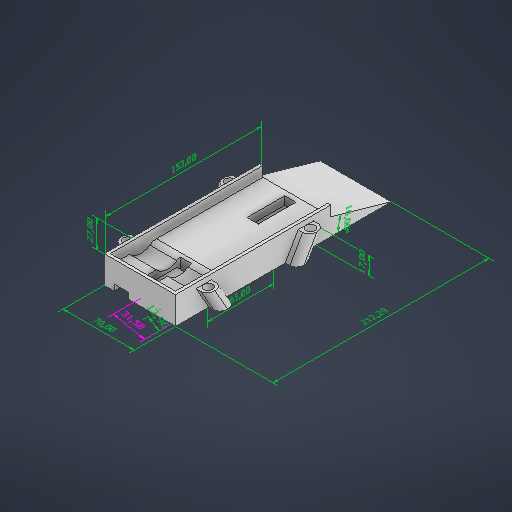
# Autodesk Inventor part: BaseCabina_v03
Saved by Autodesk Inventor 2026.1 (Build 301233020, 233B)
## iProperties
Created: 2025-10-09
Part Number: BaseCabina_v03
Material: Generic
Document SubType Name: Modeling
Designer: tito.luyo
Density: 1 g/cm^3
Appearance: Default
Author: tito.luyo
## iProperties of the stored document BaseCabina_3DPrint.ipt
Created: 2025-10-20
Part Number: BaseCabina_3DPrint
Material: Generic
Document SubType Name: Modeling
Designer: tito.luyo
Density: 1 g/cm^3
Appearance: Default
Author: tito.luyo
Autodesk Inventor part; units mm, degrees
ref_plane "YZ Plane" through (0, 0, 0) normal (1, 0, 0) x (0, 1, 0)
ref_plane "XZ Plane" through (0, 0, 0) normal (0, 1, 0) x (-1, 0, 0)
ref_plane "XY Plane" through (0, 0, 0) normal (0, 0, 1) x (1, 0, 0)
sketch "SketchBase" plane through (0, 0, 0) normal (0, 1, 0) x (-1, 0, 0)
  line L0 (0, 0) -> (70, 0)
  line L1 (70, 0) -> (70, -150)
  line L2 (70, -150) -> (0, -150)
  line L3 (0, -150) -> (0, 0)
  dimension "cabina_ancho" = 70
  dimension "cabina_largo" = 150
  constraints: 8 end point, 2 parallel, 1 horizontal, 1 perpendicular
  measures "cabina_ancho" distance of L1.end L2.end
  measures "cabina_largo" distance of L0.end L1.end
extrude "Base" add sketch "SketchBase" along normal blind 17
sketch "SketchBateria" plane through (0, 0, 0) normal (0, -1, 0) x (1, 0, 0)
  line L0 (-4, -48.5) -> (-35, -48.5)
  line L1 (-35, -48.5) -> (-35, -103.5)
  line L2 (-35, -103.5) -> (-4, -103.5)
  line L3 (-4, -103.5) -> (-4, -48.5)
  line L4 (0, 0) -> (0, -150) projected
  line L5 (-70, 0) -> (0, 0) projected
  point P0 (-19.5, -48.5)
  dimension "bateria_ancho" = 31
  dimension "bateria_largo" = 55
  dimension "bateria_sep_fondo" = 48.5
  dimension "d119" = 35
  constraints: 8 end point, 2 parallel, 1 horizontal, 1 midpoint, 1 perpendicular
  measures "bateria_ancho" distance of L2.end L1.end
  measures "bateria_largo" distance of L1.end L0.end
  measures "bateria_sep_fondo" distance from line of point (-19.5, -48.5) L5
  measures "d119" distance between parallel lines of L4 L1
extrude "Bateria" cut sketch "SketchBateria" against normal blind 7
sketch "SketchMicroControlador" plane through (0, 0, 0) normal (0, -1, 0) x (1, 0, 0)
  line L0 (-43, -5) -> (-63, -5)
  line L1 (-63, -5) -> (-63, -35)
  line L2 (-63, -35) -> (-43, -35)
  line L3 (-43, -35) -> (-43, -5)
  line L4 (-70, -150) -> (-70, 0) projected
  line L5 (-70, 0) -> (0, 0) projected
  dimension "micro_ancho" = 20
  dimension "micro_largo" = 30
  dimension "micro_sep_lateral" = 7
  dimension "micro_sep_fondo" = 5
  constraints: 8 end point, 2 parallel, 1 horizontal, 1 perpendicular
  measures "micro_ancho" distance of L2.end L1.end
  measures "micro_largo" distance of L1.end L0.end
  measures "micro_sep_lateral" distance between parallel lines of L4 L1
  measures "micro_sep_fondo" distance between parallel lines of L5 L0
extrude "MicroControlador" cut sketch "SketchMicroControlador" against normal blind 6
sketch "SketchSensorPresencia" plane through (0, 17, 0) normal (0, 1, 0) x (1, 0, 0)
  line L0 (-29.5, 108) -> (-40.5, 108)
  line L1 (-40.5, 108) -> (-40.5, 145)
  line L2 (-40.5, 145) -> (-29.5, 145)
  line L3 (-29.5, 145) -> (-29.5, 108)
  line L4 (0, 150) -> (-70, 150) projected
  line L5 (0, 0) -> (0, 150) projected
  point P0 (-35, 150)
  point P1 (-35, 145)
  dimension "presencia_ancho" = 11
  dimension "presencia_largo" = 37
  dimension "presencia_sep_fondo" = 5
  dimension "presencia_sep_lateral" = 29.5
  constraints: 8 end point, 2 midpoint, 2 parallel, 1 horizontal, 1 perpendicular
  measures "presencia_ancho" distance of L1.end L2.end
  measures "presencia_largo" distance of L0.end L1.end
  measures "presencia_sep_fondo" distance of point (-35, 150) point (-35, 145)
  measures "presencia_sep_lateral" distance between parallel lines of L5 L3
extrude "SensorPresencia" cut sketch "SketchSensorPresencia" against normal blind 8
sketch "SketchSoporte" plane through (0, 0, 0) normal (0, -1, 0) x (1, 0, 0)
  line L0 (11, -45) -> (-2, -45)
  line L1 (-2, -45) -> (-2, -30)
  line L2 (-2, -30) -> (11, -30)
  line L3 (11, -30) -> (11, -45)
  line L4 (-70, 0) -> (0, 0) projected
  line L5 (0, 0) -> (0, -150) projected
  dimension "soporte_ancho" = 13
  dimension "soporte_largo" = 15
  dimension "soporte_sep_extremo" = 30
  dimension "soporte_ins_lateral" = 11
  constraints: 8 end point, 2 parallel, 1 horizontal, 1 perpendicular
  measures "soporte_ancho" distance of L1.end L2.end
  measures "soporte_largo" distance of L0.end L1.end
  measures "soporte_sep_extremo" distance between parallel lines of L2 L4
  measures "soporte_ins_lateral" distance between parallel lines of L5 L3
sketch "SketchSoporteGuiaInclinada" plane through (0, 0, 0) normal (1, 0, 0) x (0, 0, -1)
  line L0 (150, 0) -> (0, 0) projected
  line L1 (20, 0) -> (7.2983, 22)
  dimension "soporte_guia_sep_extremo" = 20
  dimension "soporte_guia_inclinacion" = 60
  dimension "soporte_guia_altura" = 22
  constraints: 2 end point, 1 point on line
  measures "soporte_guia_sep_extremo" distance of L0.end L1.start
  measures "soporte_guia_inclinacion" angle of L0 L1
  measures "soporte_guia_altura" distance from line of L0 L1.end
sweep "Soporte" add profiles "SketchSoporte" path "SketchSoporteGuiaInclinada" path curves L1
sketch "SketchSoporteHueco" plane through (-2, 22, -17.2983) normal (0, 1, 0) x (1, 0, 0)
  circle A0 centre (6.5, 7.5) radius 4.45
  line L0 (13, 15) -> (0, 15) projected
  line L1 (0, 15) -> (0, 0) projected
  point P0 (2, -17.2983)
  dimension "soporte_hueco_diametro" = 8.9
  dimension "soporte_hueco_sep_largo" = 7.5
  dimension "soporte_hueco_sep_ancho" = 6.5
  constraints: 1 centre point
  measures "soporte_hueco_diametro" diameter of A0
  measures "soporte_hueco_sep_largo" distance from line of L0 A0.centre
  measures "soporte_hueco_sep_ancho" distance from line of L1 A0.centre
sketch3d "3D Sketch_guia_soporteHueco"
  line L0 (11, 22, -32.2983) -> (11, 0, -45)
sweep "SoporteHueco" cut profiles "SketchSoporteHueco" path "3D Sketch_guia_soporteHueco"
sketch "SketchGuiasMitadPlano" plane through (0, 0, 0) normal (0, -1, 0) x (1, 0, 0)
  line L0 (-35, -155.1159) -> (-35, 14.8841) construction
  line L1 (-70, -150) -> (-70, 0) construction
  line L2 (14.1346, -75) -> (-95.8654, -75) construction
  line L3 (0, -150) -> (-70, -150) construction
  point P0 (0, 0)
  dimension "guia_mitad_ancho_longitud" = 170
  dimension "guia_mitad_ancho_posicion" = 35
  dimension "guia_mitad_largo_longitud" = 110
  dimension "guia_mitad_largo_posicion" = 75
  constraints: 4 end point, 1 horizontal, 1 vertical
  measures "guia_mitad_ancho_longitud" distance of L0.start L0.end
  measures "guia_mitad_ancho_posicion" distance between parallel lines of L1 L0
  measures "guia_mitad_largo_longitud" distance of L2.start L2.end
  measures "guia_mitad_largo_posicion" distance between parallel lines of L3 L2
ref_plane "Work Plane Vertical Medio" through (0, 0, -75) normal (0, 0, -1) x (-1, 0, 0)
sketch "SketchGuiaVerticalCentral" plane through (0, 0, -75) normal (0, 0, -1) x (-1, 0, 0)
  line L0 (35, 32.2596) -> (35, -17.7404)
  line L1 (70, 0) -> (70, 17) construction
  point P0 (0, 0)
  dimension "guia_centro_vertical_longitud" = 50
  dimension "guia_centro_vertical_posicion" = 35
  constraints: 2 end point, 1 vertical
  measures "guia_centro_vertical_longitud" distance of L0.start L0.end
  measures "guia_centro_vertical_posicion" distance between parallel lines of L1 L0
ref_plane "Work Plane Horiz Medio" through (-35, 0, -150) normal (-1, 0, 0) x (0, 0, 1)
mirror "SensorPresencia2" about plane through (0, 0, -75) normal (0, 0, -1) of "SensorPresencia"
sketch "SketchUsbSock" plane through (0, 0, 0) normal (0, -1, 0) x (1, 0, 0)
  line L0 (-46, -5) -> (-60, -5)
  line L1 (-60, -5) -> (-60, 0)
  line L2 (-60, 0) -> (-46, 0)
  line L3 (-46, 0) -> (-46, -5)
  line L4 (-70, -150) -> (-70, 0) projected
  line L5 (-63, -5) -> (-43, -5) projected
  point P0 (0, 0)
  point P1 (-80, -30)
  dimension "micro_usbsock_largo" = 5
  dimension "micro_usbsock_ancho" = 14
  dimension "micro_usbsock_sep_lateral" = 10
  constraints: 8 end point, 2 parallel, 1 collinear, 1 horizontal, 1 perpendicular, 1 other
  measures "micro_usbsock_largo" distance between parallel lines of L2 L0
  measures "micro_usbsock_ancho" distance between parallel lines of L1 L3
extrude "Extrusion7" cut sketch "SketchUsbSock" against normal blind 6
fillet "SoporteRedondeado1" radius 6.5 1 edges at (11, 11, -23.6491)
fillet "SoporteRedondeado2" radius 6.5 1 edges at (11, 11, -38.6491)
mirror "Mirror4" about plane through (-35, 0, -150) normal (-1, 0, 0) of "Soporte", "SoporteHueco", "SoporteRedondeado1", "SoporteRedondeado2"
mirror "Mirror5" about plane through (0, 0, -75) normal (0, 0, -1) of "SoporteHueco", "Soporte", "SoporteRedondeado2", "SoporteRedondeado1", "Mirror4"
sketch "Sketch15" plane through (0, 0, 0) normal (0, -1, 0) x (1, 0, 0)
  line L0 (-50, -117.5) -> (-65, -117.5)
  line L1 (-65, -117.5) -> (-65, -145)
  line L2 (-65, -145) -> (-50, -145)
  line L3 (-50, -145) -> (-50, -117.5)
  line L4 (0, -150) -> (-70, -150) projected
  line L5 (-70, -150) -> (-70, -120) projected
  point P0 (0, 0)
  dimension "sensordistancia_ancho" = 15
  dimension "sensordistancia_largo" = 27.5
  dimension "sensordistancia_sep_fondo" = 5
  dimension "sensordistancia_sep_lateral" = 5
  constraints: 8 end point, 2 parallel, 1 horizontal, 1 perpendicular
  measures "sensordistancia_ancho" distance of L2.end L1.end
  measures "sensordistancia_largo" distance of L1.end L0.end
  measures "sensordistancia_sep_fondo" distance between parallel lines of L4 L2
  measures "sensordistancia_sep_lateral" distance between parallel lines of L5 L1
extrude "SensorDistancia" cut sketch "Sketch15" against normal blind 6
sketch "Sketch16" plane through (0, 17, 0) normal (0, 1, 0) x (1, 0, 0)
  line L0 (-3, 0) -> (0, 0)
  line L1 (0, 0) -> (0, 150)
  line L2 (0, 150) -> (-3, 150)
  line L3 (-3, 150) -> (-3, 0)
  line L4 (0, 150) -> (-70, 150) projected
  line L5 (0, 129.815) -> (0, 150) projected
  line L6 (-70, 0) -> (0, 0) projected
  line L7 (-70, 0) -> (-67, 0)
  line L8 (-67, 0) -> (-67, 150)
  line L9 (-67, 150) -> (-70, 150)
  line L10 (-70, 150) -> (-70, 0)
  line L11 (-70, 20.185) -> (-70, 0) projected
  dimension "pared_lateral_1_ancho" = 3
  dimension "pared_lateral_2_ancho" = 3
  constraints: 16 end point, 6 collinear, 4 parallel, 2 horizontal, 2 perpendicular
  measures "pared_lateral_1_ancho" distance of L2.end L1.end
  measures "pared_lateral_2_ancho" distance of L9.end L8.end
extrude "ParedesLaterales" add sketch "Sketch16" along normal blind 10 contours L3 L2 L1 L0 | L6 L10 L4 L8
sketch "Sketch17" plane through (0, 9, 0) normal (0, 1, 0) x (1, 0, 0)
  line L0 (-29.5, 108) -> (-40.5, 108)
  line L1 (-40.5, 108) -> (-40.5, 111)
  line L2 (-40.5, 111) -> (-29.5, 111)
  line L3 (-29.5, 111) -> (-29.5, 108)
  line L4 (-29.5, 108) -> (-40.5, 108) projected
  line L5 (-29.5, 145) -> (-29.5, 108) projected
  line L6 (-40.5, 108) -> (-40.5, 145) projected
  point P0 (0, 0)
  dimension "presencia_cables_hueco_ancho" = 3
  constraints: 8 end point, 3 collinear, 2 parallel, 1 horizontal, 1 perpendicular
  measures "presencia_cables_hueco_ancho" distance of L0.end L1.end
extrude "presencia_hueco" cut sketch "Sketch17" against normal blind 9
mirror "Mirror6" about plane through (0, 0, -75) normal (0, 0, -1) of "presencia_hueco"
sketch "SketchRampa" plane through (0, 0, -120) normal (1, 0, 0) x (0, 0, -1)
  line L0 (30, 0) -> (30, 27) projected
  line L1 (30, 0) -> (89.286, 0)
  line L2 (30, 0) -> (89.286, 0) construction
  line L3 (-120, 17) -> (30, 17) projected
  line L4 (89.286, 0) -> (30, 17)
  line L5 (30, 17) -> (30, 0)
  point P0 (-120, 0)
  dimension "d89" = 0
  dimension "d129" = 16
  constraints: 8 end point, 2 horizontal, 1 collinear, 1 perpendicular
  measures "d89" distance between parallel lines of L1 L2
  measures "d129" angle of L1 L4
extrude "rampa" add sketch "SketchRampa" against normal blind 70
sketch "Sketch19" plane through (-3, 17, 0) normal (-1, 0, 0) x (0, 0, 1)
  circle A0 centre (-30, 10) radius 15
  line L0 (0, 0) -> (0, 10) projected
  point P0 (0, -17)
  dimension "huecollanta_diametro" = 30
  dimension "huecollanta_altura" = 10
  dimension "huecollanta_sep_fondo" = 30
  constraints: 1 centre point
  measures "huecollanta_diametro" diameter of A0
  measures "huecollanta_altura" vertical distance of L0.start A0.centre
  measures "huecollanta_sep_fondo" distance from line of L0 A0.centre
extrude "hueco_llanta" cut sketch "Sketch19" along normal blind 64
fillet "Fillet3" radius 11 2 edges at (-16.25, 17, -41.1803) (-53.75, 17, -41.1803)
sketch "Sketch22" plane through (0, 0, 0) normal (0, -1, 0) x (1, 0, 0)
  line L0 (-50, -139.25) -> (-48.5, -139.25)
  line L1 (-29.5, -120.25) -> (-29.5, -35)
  line L2 (-67, -38.8441) -> (-40.5, -38.8441) projected
  line L3 (-50, -117.5) -> (-50, -161)
  line L4 (-43, -35) -> (-63, -35) projected
  line L5 (-40.5, -35) -> (-40.5, -118.75)
  line L6 (-50, -128.25) -> (-50, -128.25)
  line L7 (-40.5, -42) -> (-29.5, -42)
  line L8 (-29.5, -42) -> (-29.5, -39)
  line L9 (-29.5, -39) -> (-40.5, -39)
  line L10 (-40.5, -39) -> (-40.5, -42)
  line L11 (-29.5, -42) -> (-40.5, -42) projected
  line L12 (-40.5, -42) -> (-40.5, -39) projected
  line L13 (-40.5, -39) -> (-29.5, -39) projected
  line L14 (-40.5, -111) -> (-29.5, -111)
  line L15 (-29.5, -111) -> (-29.5, -108)
  line L16 (-29.5, -108) -> (-40.5, -108)
  line L17 (-40.5, -108) -> (-40.5, -111)
  line L18 (-29.5, -111) -> (-40.5, -111) projected
  line L19 (-40.5, -111) -> (-40.5, -108) projected
  line L20 (-40.5, -108) -> (-29.5, -108) projected
  line L21 (-29.5, -35) -> (-29.5, -21.3)
  line L22 (-29.5, -21.3) -> (-43, -21.3)
  line L23 (-43, -5) -> (-43, -35) projected
  line L24 (-40.5, -35) -> (-43, -35)
  line L25 (-65, -117.5) -> (-50, -117.5) projected
  arc A0 (-50, -128.25) -> (-40.5, -118.75) centre (-50, -118.75) ccw
  arc A1 (-48.5, -139.25) -> (-29.5, -120.25) centre (-48.5, -120.25) ccw
  point P0 (0, 0)
  point P1 (-29.5, -139.25)
  point P2 (-40.5, -128.25)
  point P3 (-35, -42)
  point P4 (-35, -39)
  point P5 (-40.5, -111)
  point P6 (-40.5, -108)
  point P7 (-40.5, -42)
  point P8 (-40.5, -39)
  dimension "d112" = 11
  dimension "d120" = 13.7
  dimension "d167" = 21.75
  dimension "d168" = 20.5
  dimension "d196" = 9.5
  dimension "d197" = 19
  constraints: 32 end point, 8 collinear, 5 point on line, 4 horizontal, 4 parallel, 4 perpendicular, 4 point on circle, 4 tangent, 2 centre point, 1 midpoint, 1 vertical, 3 other
  measures "d112" distance between parallel lines of L1 L5
  measures "d120" distance of L1.end L21.end
  measures "d167" distance between parallel lines of L25 L0
  measures "d168" distance between parallel lines of L3 L1
  measures "d196" radius of A0
  measures "d197" radius of A1
extrude "canaleta_central" cut sketch "Sketch22" against normal blind 6
sketch "Sketch24" plane through (-46, 0, 0) normal (0, 0, 1) x (1, 0, 0)
  line L0 (-28.5, 22) -> (-24, 22) projected
  line L1 (-24, 0) -> (-28.5, 0) projected
  line L2 (-14, 0) -> (-14, 6) projected
  line L3 (-24, 0) -> (-14, 0)
  line L4 (-14, 0) -> (-14, 6)
  line L5 (-14, 6) -> (0, 6) projected
  line L6 (-14, 6) -> (0, 6)
  line L7 (0, 6) -> (0, 0)
  line L8 (46, 0) -> (50.5, 0) projected
  line L9 (0, 0) -> (46, 0)
  line L10 (-24, 22) -> (-24, 0) projected
  line L11 (-21, 27) -> (-24, 27) projected
  line L12 (-24, 0) -> (-24, 27)
  line L13 (46, 0) -> (46, 27) projected
  line L14 (-24, 27) -> (46, 27)
  line L15 (46, 27) -> (46, 0)
  point P0 (-21.5, 22)
  constraints: 16 end point, 4 perpendicular, 3 collinear, 1 point on line, 1 vertical
extrude "pared_fondo" add sketch "Sketch24" along normal blind 3
sketch "Sketch25" plane through (0, 0, 0) normal (0, -1, 0) x (1, 0, 0)
  line L0 (-4, -20.5) -> (-43, -20.5)
  line L1 (-43, -20.5) -> (-43, -5)
  line L2 (-43, -5) -> (-4, -5)
  line L3 (-4, -5) -> (-4, -20.5)
  line L4 (-43, -5) -> (-43, -21.3) projected
  line L5 (-46, -5) -> (-43, -5) projected
  line L6 (-4, -48.5) -> (-4, -103.5) projected
  line L7 (-4, -20.5) -> (-9, -20.5)
  line L8 (-9, -20.5) -> (-9, -48.5)
  line L9 (-9, -48.5) -> (-4, -48.5)
  line L10 (-4, -48.5) -> (-4, -20.5)
  line L11 (-29.5, -48.5) -> (-4, -48.5) projected
  point P0 (0, 0)
  point P1 (-43, -35)
  dimension "d122" = 15.5
  dimension "d123" = 5
  constraints: 16 end point, 4 collinear, 4 parallel, 2 horizontal, 2 perpendicular
  measures "d122" distance of L0.end L1.end
  measures "d123" distance of L9.end L8.end
extrude "BEC" cut sketch "Sketch25" against normal blind 6
sketch "Sketch26" plane through (0, 0, 0) normal (0, -1, 0) x (1, 0, 0)
  circle A0 centre (-15, -43.5) radius 1.85
  line L0 (0, -45) -> (0, -105) projected
  line L1 (-29.5, -48.5) -> (-9, -48.5) projected
  point P0 (0, 0)
  dimension "d145" = 3.7
  dimension "d146" = 15
  dimension "d147" = 5
  constraints: 1 centre point
  measures "d145" diameter of A0
  measures "d146" distance from line of A0.centre L0
  measures "d147" distance from line of L1 A0.centre
extrude "Extrusion18" cut sketch "Sketch26" against normal blind 6.85
sketch "Sketch27" plane through (0, 0, 0) normal (0, -1, 0) x (1, 0, 0)
  circle A0 centre (-15, -43.5) radius 1.85 projected
  circle A1 centre (-15, -43.5) radius 1.95
  point P0 (0, 0)
  dimension "d150" = 3.9
  constraints: 1 centre point, 1 coincident
  measures "d150" diameter of A1
extrude "Extrusion19" cut sketch "Sketch27" against normal blind 2
sketch "Sketch28" plane through (0, 0, 0) normal (0, -1, 0) x (1, 0, 0)
  circle A0 centre (-15, -108.5) radius 1.85
  line L0 (0, -45) -> (0, -105) projected
  line L1 (-4, -103.5) -> (-29.5, -103.5) projected
  point P0 (0, 0)
  dimension "d153" = 3.7
  dimension "d154" = 15
  dimension "d155" = 5
  constraints: 1 centre point
  measures "d153" diameter of A0
  measures "d154" distance from line of L0 A0.centre
  measures "d155" distance from line of L1 A0.centre
extrude "Extrusion20" cut sketch "Sketch28" against normal blind 6.85
sketch "Sketch29" plane through (0, 0, 0) normal (0, -1, 0) x (1, 0, 0)
  circle A0 centre (-15, -108.5) radius 1.85 projected
  circle A1 centre (-15, -108.5) radius 1.95
  point P0 (0, 0)
  dimension "d158" = 3.9
  constraints: 1 centre point, 1 coincident
  measures "d158" diameter of A1
extrude "Extrusion21" cut sketch "Sketch29" against normal blind 2
sketch "Sketch30" plane through (0, 6, 0) normal (0, -1, 0) x (1, 0, 0)
  line L0 (-40.5, -35) -> (-63, -35) projected
  line L1 (-42.6, -35) -> (-42.6, -35)
  line L2 (-42.2, -34.6) -> (-42.2, -5.4)
  line L3 (-42.6, -5) -> (-42.6, -5)
  line L4 (-43, -5.4) -> (-43, -34.6)
  line L5 (-43, -20.5) -> (-43, -21.3) projected
  line L6 (-50, -139.25) -> (-50, -145) projected
  line L7 (-49.6, -139.25) -> (-49.6, -139.25)
  line L8 (-49.2, -138.85) -> (-49.2, -128.65)
  line L9 (-49.6, -128.25) -> (-49.6, -128.25)
  line L10 (-50, -128.65) -> (-50, -138.85)
  line L11 (-35.4, -108) -> (-35.4, -108)
  line L12 (-35, -107.6) -> (-35, -42.4)
  line L13 (-35.4, -42) -> (-35.4, -42)
  line L14 (-35.8, -42.4) -> (-35.8, -107.6)
  line L15 (-29.5, -108) -> (-40.5, -108) projected
  line L16 (-40.5, -42) -> (-29.5, -42) projected
  line L17 (-35, -48.5) -> (-35, -103.5) projected
  line L18 (-40.5, -118.75) -> (-40.5, -35) projected
  line L19 (-9, -48.5) -> (-9, -20.5) projected
  line L20 (-8.6, -20.5) -> (-4.4, -20.5)
  line L21 (-4, -20.9) -> (-4, -20.9)
  line L22 (-4.4, -21.3) -> (-8.6, -21.3)
  line L23 (-9, -20.9) -> (-9, -20.9)
  line L24 (-9, -20.5) -> (-43, -20.5) projected
  line L25 (-33.2, -20.5) -> (-33.2, -20.5)
  line L26 (-32.8, -20.1) -> (-32.8, -5.4)
  line L27 (-33.2, -5) -> (-33.2, -5)
  line L28 (-33.6, -5.4) -> (-33.6, -20.1)
  line L29 (-10.4, -20.5) -> (-10.4, -20.5)
  line L30 (-10.8, -20.1) -> (-10.8, -5.4)
  line L31 (-10.4, -5) -> (-10.4, -5)
  line L32 (-10, -5.4) -> (-10, -20.1)
  line L33 (-4, -5) -> (-4, -103.5) projected
  arc A0 (-10.8, -20.1) -> (-10.4, -20.5) centre (-10.4, -20.1) ccw
  arc A1 (-10.4, -20.5) -> (-10, -20.1) centre (-10.4, -20.1) ccw
  arc A2 (-10, -5.4) -> (-10.4, -5) centre (-10.4, -5.4) ccw
  arc A3 (-10.4, -5) -> (-10.8, -5.4) centre (-10.4, -5.4) ccw
  arc A4 (-9, -20.9) -> (-8.6, -21.3) centre (-8.6, -20.9) ccw
  arc A5 (-8.6, -20.5) -> (-9, -20.9) centre (-8.6, -20.9) ccw
  arc A6 (-4.4, -21.3) -> (-4, -20.9) centre (-4.4, -20.9) ccw
  arc A7 (-4, -20.9) -> (-4.4, -20.5) centre (-4.4, -20.9) ccw
  arc A8 (-33.6, -20.1) -> (-33.2, -20.5) centre (-33.2, -20.1) ccw
  arc A9 (-33.2, -20.5) -> (-32.8, -20.1) centre (-33.2, -20.1) ccw
  arc A10 (-33.2, -5) -> (-33.6, -5.4) centre (-33.2, -5.4) ccw
  arc A11 (-32.8, -5.4) -> (-33.2, -5) centre (-33.2, -5.4) ccw
  arc A12 (-42.6, -5) -> (-43, -5.4) centre (-42.6, -5.4) ccw
  arc A13 (-42.2, -5.4) -> (-42.6, -5) centre (-42.6, -5.4) ccw
  arc A14 (-43, -34.6) -> (-42.6, -35) centre (-42.6, -34.6) ccw
  arc A15 (-42.6, -35) -> (-42.2, -34.6) centre (-42.6, -34.6) ccw
  arc A16 (-35, -42.4) -> (-35.4, -42) centre (-35.4, -42.4) ccw
  arc A17 (-35.4, -42) -> (-35.8, -42.4) centre (-35.4, -42.4) ccw
  arc A18 (-35.4, -108) -> (-35, -107.6) centre (-35.4, -107.6) ccw
  arc A19 (-35.8, -107.6) -> (-35.4, -108) centre (-35.4, -107.6) ccw
  arc A20 (-49.6, -128.25) -> (-50, -128.65) centre (-49.6, -128.65) ccw
  arc A21 (-49.2, -128.65) -> (-49.6, -128.25) centre (-49.6, -128.65) ccw
  arc A22 (-50, -138.85) -> (-49.6, -139.25) centre (-49.6, -138.85) ccw
  arc A23 (-49.6, -139.25) -> (-49.2, -138.85) centre (-49.6, -138.85) ccw
  line L34 (-35.8, -86.4) -> (-40.1, -86.4)
  line L35 (-40.5, -86) -> (-40.5, -86)
  line L36 (-40.1, -85.6) -> (-35.8, -85.6)
  line L37 (-35.8, -85.6) -> (-35.8, -86.4)
  line L38 (-35.8, -64.4) -> (-40.1, -64.4)
  line L39 (-40.5, -64) -> (-40.5, -64)
  line L40 (-40.1, -63.6) -> (-35.8, -63.6)
  line L41 (-35.8, -63.6) -> (-35.8, -64.4)
  arc A24 (-40.5, -86) -> (-40.1, -86.4) centre (-40.1, -86) ccw
  arc A25 (-40.1, -85.6) -> (-40.5, -86) centre (-40.1, -86) ccw
  arc A26 (-40.5, -64) -> (-40.1, -64.4) centre (-40.1, -64) ccw
  arc A27 (-40.1, -63.6) -> (-40.5, -64) centre (-40.1, -64) ccw
  point P0 (0, 0)
  point P1 (-43, -35)
  point P2 (-42.2, -5)
  point P3 (-42.2, -35)
  point P4 (-43, -5)
  point P5 (-49.2, -128.25)
  point P6 (-49.2, -139.25)
  point P7 (-50, -128.25)
  point P8 (-35.8, -108)
  point P9 (-35, -42)
  point P10 (-35, -108)
  point P11 (-35.8, -42)
  point P12 (-4, -21.3)
  point P13 (-4, -20.5)
  point P14 (-9, -21.3)
  point P15 (-9, -21.3)
  point P16 (-42.2, -35)
  point P17 (-33.6, -20.5)
  point P18 (-32.8, -5)
  point P19 (-32.8, -20.5)
  point P20 (-33.6, -5)
  point P21 (-32.8, -20.5)
  point P22 (-10, -20.5)
  point P23 (-10.8, -5)
  point P24 (-10.8, -20.5)
  point P25 (-10, -5)
  point P26 (-10.8, -20.5)
  point P27 (-40.5, -85.6)
  point P28 (-40.5, -86.4)
  point P29 (-40.5, -63.6)
  point P30 (-40.5, -64.4)
  point P31 (-40.5, -64)
  point P32 (-40.5, -64)
  dimension "d169" = 0.8
  dimension "d170" = 30
  dimension "d171" = 0.8
  dimension "d172" = 11
  dimension "d173" = 0.8
  dimension "d176" = 5
  dimension "d177" = 0.8
  dimension "d180" = 0.8
  dimension "d181" = 15.5
  dimension "d183" = 0.8
  dimension "d184" = 15.5
  dimension "d185" = 22
  dimension "d186" = 6
  dimension "d187" = 0.4
  dimension "d188" = 4.7
  dimension "d189" = 0.8
  dimension "d190" = 4.7
  dimension "d191" = 0.8
  dimension "d192" = 22
  dimension "d193" = 22
  dimension "d194" = 0.4
  dimension "d195" = 0.4
  constraints: 64 end point, 61 point on line, 56 point on circle, 56 tangent, 28 centre point, 25 equal radius, 16 parallel, 8 horizontal, 8 perpendicular, 4 collinear, 2 midpoint
  measures "d169" distance of point (-43, -5) point (-42.2, -5)
  measures "d170" distance of point (-42.2, -5) point (-42.2, -35)
  measures "d171" distance of point (-50, -128.25) point (-49.2, -128.25)
  measures "d172" distance of point (-49.2, -128.25) point (-49.2, -139.25)
  measures "d173" distance of point (-35.8, -42) point (-35, -42)
  measures "d176" distance of point (-4, -21.3) point (-9, -21.3)
  measures "d177" distance of point (-4, -20.5) point (-4, -21.3)
  measures "d180" distance of point (-33.6, -5) point (-32.8, -5)
  measures "d181" distance of point (-32.8, -5) point (-32.8, -20.5)
  measures "d183" distance of point (-10.8, -5) point (-10, -5)
  measures "d184" distance of point (-10.8, -20.5) point (-10.8, -5)
  measures "d185" distance between parallel lines of L26 L30
  measures "d186" distance between parallel lines of L32 L33
  measures "d187" radius of A0
  measures "d188" distance of point (-40.5, -85.6) L36.end
  measures "d189" distance of point (-40.5, -86.4) point (-40.5, -85.6)
  measures "d190" distance of point (-40.5, -63.6) L40.end
  measures "d191" distance of point (-40.5, -64.4) point (-40.5, -63.6)
  measures "d192" distance from line of L15 point (-40.5, -86)
  measures "d193" distance of point (-40.5, -64) point (-40.5, -86)
  measures "d194" radius of A24
  measures "d195" radius of A26
extrude "soportes" add sketch "Sketch30" along normal blind 6 contours A15 A14 L4 L24 L2 | L24 L4 A12 A13 L2 | A23 A22 L10 A20 A21 L8 | A18 A19 L14 A17 A16 L12 | A25 L36 L14 L34 A24 | A27 L40 L14 L38 A26 | L20 A7 A6 L22 A4 A5 | A9 A8 L28 A10 A11 L26 | L30 A3 A2 L32 A1 A0
equation "\"presencia_sep_lateral\" = -0.5 * presencia_ancho + 0.5 * cabina_ancho"
equation "\"soporte_hueco_sep_largo\" = 0.5 * soporte_largo"
equation "\"soporte_hueco_sep_ancho\" = 0.5 * soporte_ancho"
equation "\"guia_mitad_ancho_posicion\" = 0.5 * cabina_ancho"
equation "\"guia_mitad_largo_posicion\" = 0.5 * cabina_largo"
equation "\"guia_centro_vertical_posicion\" = 0.5 * cabina_ancho"
equation "\"micro_usbsock_largo\" = micro_sep_fondo"
equation "\"micro_usbsock_sep_lateral\" = micro_sep_lateral + 0.5 * micro_ancho - 0.5 * micro_usbsock_ancho"
equation "\"micro_usbsock_espesor\" = micro_espesor"
equation "\"soporte_redondeado2\" = soporte_redondeado1"
equation "\"presencia_cables_hueco_espesor\" = cabina_espesor - presencia_espesor"
equation "\"rampa_ancho\" = cabina_ancho"
equation "\"huecollanta_ancho\" = -pared_lateral_1_ancho + cabina_ancho - pared_lateral_2_ancho"
equation "\"d112\" = ranura_ancho"
equation "\"llantas_distancia_ejes\" = 89"
equation "\"llantas_distancia_ancho\" = 47"
equation "\"llantas_ancho\" = 8.5"
equation "\"llantas_diametro\" = 25.6"
equation "\"soporte_hueco_tolerancia\" = 0.9"
equation "\"micro_espesor\" = 6"
equation "\"soporte_redondeado1\" = 6.5"
equation "\"cabina_espesor\" = 17"
equation "\"presencia_espesor\" = 8"
equation "\"ranura_ancho\" = 11"
body "Solid1"
